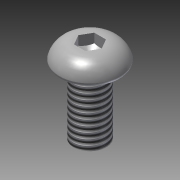
# Autodesk Inventor part: screw_M3_10_hex
Saved by Autodesk Inventor 2013 (Build 170138000, 138)
## iProperties
Shininess: 50.0
Created: 2012-07-28
Part Number: screw_M3_10_hex
Document SubType Name: Modeling
Designer: Noa Izumi
Material: Default
Density: 1 g/cm^3
Density: 0.0
Volumn: 0.0
Area: 0.0
PropertySet Name: Model Information
Control State: 0
Master: False
Checked Out: False
Author: Noa Izumi
Autodesk Inventor part; units mm, degrees
ref_plane "YZ Plane" through (0, 0, 0) normal (1, 0, 0) x (0, 1, 0)
ref_plane "XZ Plane" through (0, 0, 0) normal (0, 1, 0) x (-1, 0, 0)
ref_plane "XY Plane" through (0, 0, 0) normal (0, 0, 1) x (1, 0, 0)
sketch "Sketch1" plane through (0, 0, 0) normal (0, 0, 1) x (1, 0, 0)
  circle A0 centre (0, 0) radius 3.75
  dimension "d0" = 7.5
  constraints: 1 centre point
  measures "d0" diameter of A0
extrude "Extrusion1" add sketch "Sketch1" along normal blind 2.3
fillet "Fillet3" radius 0.5 1 edges at (-3.75, 0, 0)
fillet "Fillet4" radius 2.3 1 edges at (-3.75, 0, 2.3)
sketch "草圖6" plane through (0, 0, 2.3) normal (0, 0, 1) x (1, 0, 0)
  circle A0 centre (0, 0) radius 1.505 projected
  line L0 (0.7217, 1.25) -> (1.4434, 0)
  line L1 (1.4434, 0) -> (0.7217, -1.25)
  line L2 (0.7217, -1.25) -> (-0.7217, -1.25)
  line L3 (-0.7217, -1.25) -> (-1.4434, 0)
  line L4 (-1.4434, 0) -> (-0.7217, 1.25)
  line L5 (-0.7217, 1.25) -> (0.7217, 1.25)
  dimension "d27" = 2.5
  constraints: 12 end point, 1 coincident, 13 other
  measures "d27" distance between parallel lines of L2 L5
extrude "擠出4" cut sketch "草圖6" against normal blind 2 contours L0 L1 L2 L3 L4 L5
sketch "草圖7" plane through (0, 0, 0) normal (1, 0, 0) x (0, 1, 0)
  line L0 (0, 0.3) -> (-2, 1.5017)
  line L1 (-2, 1.5017) -> (-2, 0.3)
  line L2 (0, 0.3) -> (-2, 0.3)
  line L3 (0, 0) -> (0, 2.4201)
  dimension "d30" = 0.3
  dimension "d31" = 31
  dimension "d34" = 2
  constraints: 8 end point, 2 perpendicular, 1 vertical
  measures "d30" distance of L3.start L0.start
  measures "d31" angle of L2 L0
  measures "d34" distance of L0.start L1.end
revolve "迴轉3" add sketch "草圖7" angle 360 about axis through (0, 0, 0) along (0, 0, 1)
sketch "草圖8" plane through (0, 0, 0) normal (0, 0, -1) x (-1, 0, 0)
  circle A0 centre (0, 0) radius 3.25 projected
  circle A1 centre (0, 0) radius 2
  dimension "d35" = 4
  constraints: 1 centre point, 1 coincident
  measures "d35" diameter of A1
extrude "擠出5" add sketch "草圖8" along normal blind 8 contours A1
thread "螺紋2" size "M4x0.7" class "6g" standard "ANSI Metric M Profile" full length
